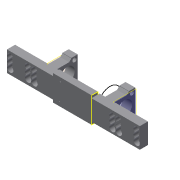
# Autodesk Inventor part: 20_Base_STORMchip_doublesided
Saved by Autodesk Inventor 2019 (Build 230136000, 136)
## iProperties
Created: 2018-09-25
Part Number: 20_Base_STORMchip_doublesided
Material: Generic
Document SubType Name: Modeling
Designer: diederichbenedict
Density: 1 g/cm^3
Appearance: Default
Author: diederichbenedict
Autodesk Inventor part; units mm, degrees
ref_plane "YZ Plane" through (0, 0, 0) normal (1, 0, 0) x (0, 1, 0)
ref_plane "XZ Plane" through (0, 0, 0) normal (0, 1, 0) x (-1, 0, 0)
ref_plane "Work Plane1" through (0, 0, 40) normal (0, 0, 1) x (1, 0, 0)
sketch "Sketch1" plane through (0, 0, 40) normal (0, 0, 1) x (1, 0, 0)
  circle A0 centre (-3.7974, 17.669) radius 1.2295 construction
  line L0 (-20.6474, 15.7142) -> (-23.4129, 15.7142) construction
  arc A1 (-23.4129, 15.7142) -> (-23.682, 15.7142) centre (-23.5474, 13.819) ccw construction
  line L1 (-23.682, 15.7142) -> (-26.0625, 15.7142) construction
  arc A2 (-24.2285, 17.7142) -> (-26.0625, 15.7142) centre (-6.7472, -0.1577) ccw construction
  line L2 (-24.2285, 17.7142) -> (-26.3758, 17.7142) construction
  arc A3 (-26.3758, 17.7142) -> (-24.7023, 19.2398) centre (-27.9474, 21.119) ccw construction
  line L3 (-24.7023, 19.2398) -> (-24.6974, 19.2426) construction
  line L4 (-24.6974, 19.2426) -> (-24.6974, 19.2481) construction
  arc A4 (-24.6974, 19.2481) -> (-24.2285, 20.6377) centre (-27.9474, 21.119) ccw construction
  line L5 (-24.2285, 20.6377) -> (-24.2285, 21.6002) construction
  arc A5 (-24.2285, 21.6002) -> (-24.6974, 22.9898) centre (-27.9474, 21.119) ccw construction
  line L6 (-24.6974, 22.9898) -> (-24.6974, 22.9953) construction
  line L7 (-24.6974, 22.9953) -> (-24.7023, 22.9981) construction
  arc A6 (-24.7023, 22.9981) -> (-24.7753, 23.119) centre (-27.9474, 21.119) ccw construction
  line L8 (-24.2285, 23.119) -> (-24.7753, 23.119) construction
  line L9 (-24.2285, 23.119) -> (-24.2285, 25.119) construction
  line L10 (13.224, 25.119) -> (-24.2285, 25.119) construction
  line L11 (13.224, 15.7142) -> (13.224, 25.119) construction
  line L12 (13.224, 15.7142) -> (24.5758, 15.7142) construction
  line L13 (24.5758, 15.7142) -> (24.5758, 9.2277) construction
  line L14 (24.5758, 9.2277) -> (27.1274, 9.2277) construction
  arc A7 (27.1274, 9.2277) -> (29.8148, 4.5037) centre (29.5758, 7.4941) ccw construction
  line L15 (29.8148, 4.5037) -> (29.8148, 2.9857) construction
  arc A8 (29.8148, 2.9857) -> (29.8148, -2.9952) centre (29.5758, -0.0048) ccw construction
  line L16 (29.8148, -2.9952) -> (29.8148, -5.513) construction
  arc A9 (29.8148, -5.513) -> (27.1391, -10.2535) centre (29.5758, -8.5035) ccw construction
  line L17 (27.1391, -10.2535) -> (24.5758, -10.2535) construction
  line L18 (24.5758, -10.2535) -> (24.5758, -16.281) construction
  line L19 (24.5758, -16.281) -> (13.5758, -16.281) construction
  line L20 (13.5758, -16.281) -> (13.5758, -24.681) construction
  line L21 (-15.9474, -24.681) -> (13.5758, -24.681) construction
  line L22 (-15.9474, -24.681) -> (-15.9474, -23.4032) construction
  arc A10 (-17.9474, -22.5084) -> (-15.9474, -23.4032) centre (-6.7472, -0.1577) ccw construction
  line L23 (-17.9474, -22.5084) -> (-17.9474, -22.681) construction
  line L24 (-24.7753, -22.681) -> (-17.9474, -22.681) construction
  arc A11 (-24.7753, -22.681) -> (-24.7023, -22.5602) centre (-27.9474, -20.681) ccw construction
  line L25 (-24.7023, -22.5602) -> (-24.6974, -22.5574) construction
  line L26 (-24.6974, -22.5574) -> (-24.6974, -22.5519) construction
  arc A12 (-24.6974, -22.5519) -> (-24.6974, -18.8102) centre (-27.9474, -20.681) ccw construction
  line L27 (-24.6974, -18.8102) -> (-24.6974, -18.8047) construction
  line L28 (-24.6974, -18.8047) -> (-24.7023, -18.8019) construction
  arc A13 (-24.7023, -18.8019) -> (-26.3655, -17.281) centre (-27.9474, -20.681) ccw construction
  line L29 (-26.3655, -17.281) -> (-27.3364, -17.281) construction
  line L30 (-27.3364, -17.281) -> (-27.9474, -16.9283) construction
  line L31 (-28.2786, -17.1195) -> (-27.9474, -16.9283) construction
  line L32 (-28.2786, -17.1195) -> (-28.2786, -16.9457) construction
  arc A14 (-28.2786, -16.9457) -> (-29.9474, -17.5089) centre (-27.9474, -20.681) ccw construction
  line L33 (-29.9474, -14.281) -> (-29.9474, -17.5089) construction
  line L34 (-72.9474, -14.281) -> (-29.9474, -14.281) construction
  line L35 (-72.9474, -12.281) -> (-72.9474, -14.281) construction
  arc A15 (-72.9474, -12.281) -> (-66.9474, -4.281) centre (-69.9474, -8.281) ccw construction
  arc A16 (-66.9474, -4.281) -> (-66.9474, 3.719) centre (-69.9474, -0.281) ccw construction
  arc A17 (-66.9474, 3.719) -> (-72.9474, 11.719) centre (-69.9474, 7.719) ccw construction
  line L36 (-72.9474, 13.7142) -> (-72.9474, 11.719) construction
  line L37 (-29.9474, 13.7142) -> (-72.9474, 13.7142) construction
  line L38 (-29.9474, 17.9468) -> (-29.9474, 13.7142) construction
  arc A18 (-29.9474, 17.9468) -> (-28.9474, 17.5047) centre (-27.9474, 21.119) ccw construction
  line L39 (-28.9474, 17.5047) -> (-28.9474, 12.719) construction
  line L40 (-28.9474, 12.719) -> (-28.1759, 12.719) construction
  arc A19 (-26.9474, 14.5715) -> (-28.1759, 12.719) centre (-6.7472, -0.1577) ccw construction
  line L41 (-26.9474, 14.5715) -> (-26.9474, 15.7142) construction
  line L42 (-26.9474, 15.7142) -> (-26.0625, 15.7142) construction
  line L43 (-26.0625, 15.7142) -> (-26.0625, 11.2745) construction
  line L44 (-26.0625, 11.2745) -> (-20.6474, 11.2745) construction
  line L45 (-20.6474, 11.2745) -> (-20.6474, 15.7142) construction
  line L46 (-19.9474, -11.731) -> (-23.1888, -11.731) construction
  arc A20 (-23.1888, -11.731) -> (-25.6444, -11.731) centre (-24.4166, -13.181) ccw construction
  line L47 (-25.6444, -11.731) -> (-27.3166, -11.731) construction
  line L48 (-27.3166, -11.731) -> (-27.3166, -16.481) construction
  line L49 (-27.3166, -16.481) -> (-19.9474, -16.481) construction
  line L50 (-19.9474, -16.481) -> (-19.9474, -11.731) construction
  arc A21 (-24.2786, -17.9803) -> (-22.8499, -19.281) centre (-6.7472, -0.1577) ccw construction
  line L51 (-24.2786, -19.281) -> (-24.2786, -17.9803) construction
  line L52 (-24.2786, -19.281) -> (-22.8499, -19.281) construction
  circle A22 centre (-48.8966, -9.0098) radius 1.45 construction
  circle A23 centre (-62.8966, 8.9902) radius 1.45 construction
  circle A24 centre (-55.8966, -0.0098) radius 1.45 construction
  circle A25 centre (-48.8966, 8.9902) radius 1.45 construction
  circle A26 centre (-62.8966, -9.0098) radius 1.45 construction
  arc A27 (-29.7867, -9.8622) -> (-28.8998, -11.7448) centre (-6.7472, -0.1577) ccw construction
  arc A28 (-29.7867, -9.8622) -> (-31.3026, -4.8512) centre (-31.9474, -7.781) ccw construction
  arc A29 (-31.5545, -3.2552) -> (-31.3026, -4.8512) centre (-6.7472, -0.1577) ccw construction
  arc A30 (-31.5545, -3.2552) -> (-31.5837, 2.6968) centre (-31.9474, -0.281) ccw construction
  arc A31 (-31.1373, 5.3304) -> (-31.5837, 2.6968) centre (-6.7472, -0.1577) ccw construction
  arc A32 (-31.1373, 5.3304) -> (-29.5693, 10.0477) centre (-31.9474, 8.219) ccw construction
  arc A33 (-28.6194, 11.9504) -> (-29.5693, 10.0477) centre (-6.7472, -0.1577) ccw construction
  arc A34 (-28.6194, 11.9504) -> (-36.9474, 8.219) centre (-31.9474, 8.219) ccw construction
  arc A35 (-36.9474, 8.219) -> (-44.5814, 3.969) centre (-41.9474, 8.219) ccw construction
  arc A36 (-44.5814, 3.969) -> (-45.2546, -4.031) centre (-41.9474, -0.281) ccw construction
  arc A37 (-45.2546, -4.031) -> (-36.9474, -7.781) centre (-41.9474, -7.781) ccw construction
  arc A38 (-36.9474, -7.781) -> (-28.8998, -11.7448) centre (-31.9474, -7.781) ccw construction
  line L53 (-19.9474, -11.731) -> (-27.3166, -11.731) construction
  line L54 (-27.3166, -11.731) -> (-27.3166, -16.481) construction
  line L55 (-27.3166, -16.481) -> (-19.9474, -16.481) construction
  line L56 (-19.9474, -16.481) -> (-19.9474, -11.731) construction
  line L57 (-20.6474, 11.2745) -> (-27.3166, 11.2745) construction
  line L58 (-27.3166, 11.2745) -> (-27.3166, 15.7142) construction
  line L59 (-27.3166, 15.7142) -> (-20.6474, 15.7142) construction
  line L60 (-20.6474, 15.7142) -> (-20.6474, 11.2745) construction
  line L61 (-19.9474, -16.481) -> (-27.3166, -16.481)
  line L62 (-27.3166, -16.481) -> (-27.3166, -11.731)
  line L63 (-27.3166, -11.731) -> (-19.9474, -11.731)
  line L64 (-19.9474, -11.731) -> (-19.9474, -16.481)
  line L65 (-20.6474, 11.2745) -> (-27.3166, 11.2745)
  line L66 (-27.3166, 11.2745) -> (-27.3166, 15.7142)
  line L67 (-27.3166, 15.7142) -> (-20.6474, 15.7142)
  line L68 (-20.6474, 15.7142) -> (-20.6474, 11.2745) construction
  circle A39 centre (-24.4166, -13.181) radius 0.6105 projected
  circle A40 centre (-24.4166, -13.181) radius 0.9 projected
  circle A41 centre (-23.5474, 13.819) radius 0.9 projected
  line L69 (-27.3166, -11.731) -> (-21.5681, -11.731)
  line L70 (-21.5681, -11.731) -> (-21.5681, -15.2316)
  line L71 (-21.5681, -15.2316) -> (-27.3166, -15.2316)
  line L72 (-27.3166, -15.2316) -> (-27.3166, -11.731)
  line L73 (-21.5681, 15.7142) -> (-21.5681, 12.3429)
  line L74 (-21.5681, 12.3429) -> (-22.6365, 11.2745)
  point P0 (0, 0)
  dimension "d15" = 135
  constraints: 44 end point, 10 parallel, 6 perpendicular, 5 horizontal, 4 point on line
  measures "d15" angle of L73 L74
extrude "Extrusion1" add sketch "Sketch1" along normal blind 2.0006 contours L62 L63 L70 L71 | L65 L66 L67 L73 L74
sketch "Sketch3" plane through (0, 0, 42.0006) normal (0, 0, 1) x (1, 0, 0)
  line L0 (-26.1307, 11.2745) -> (-26.1307, 15.7142) projected
  line L1 (-26.1307, 15.7142) -> (-19.4616, 15.7142) projected
  line L2 (-19.4616, 15.7142) -> (-19.4616, 11.2745) projected
  line L3 (-19.4616, 11.2745) -> (-26.1307, 11.2745) projected
  line L4 (-18.7616, -11.731) -> (-26.1307, -11.731) projected
  line L5 (-18.7616, -16.481) -> (-18.7616, -11.731) projected
  line L6 (-26.1307, -16.481) -> (-18.7616, -16.481) projected
  line L7 (-26.1307, -11.731) -> (-26.1307, -16.481) projected
  line L8 (-34.5116, -20.2858) -> (-34.5116, 19.7142) projected
  line L9 (25.4884, -20.2858) -> (-34.5116, -20.2858) projected
  line L10 (25.4884, 19.7142) -> (25.4884, -20.2858) projected
  line L11 (-34.5116, 19.7142) -> (25.4884, 19.7142) projected
  circle A0 centre (-24.4166, -13.181) radius 0.9 projected
  circle A1 centre (-23.5474, 13.819) radius 0.9 projected
  point P0 (0, 0)
extrude "Extrusion3" add sketch "Sketch3" along normal blind 10 contours L0 L1 L2 L3 | L5 L6 L7 L4 | L8 L11 L10 L9
sketch "Sketch4" plane through (25.4884, -20.2858, 42.0006) normal (1, 0, 0) x (0, 0, -1)
  line L0 (0, 0) -> (0, 40) projected
  line L1 (0, 40) -> (-10, 40) projected
  line L2 (-10, 0) -> (-10, 40) projected
  line L3 (0, 0) -> (-10, 0) projected
  circle A0 centre (18.7347, 20) radius 17.8578
  point P0 (42.0006, 20.2858)
  constraints: 1 centre point
sketch "Sketch5" plane through (0, 0, 42.0006) normal (0, 0, -1) x (-1, 0, 0)
  circle A0 centre (-22.3026, 2.519) radius 0.6105 projected
  line L0 (-20.5026, 4.519) -> (-24.3026, 4.519) projected
  line L1 (-24.3026, 4.519) -> (-24.3026, -2.881) projected
  line L2 (-24.3026, -2.881) -> (-20.5026, -2.881) projected
  line L3 (-20.5026, -2.881) -> (-20.5026, 4.519) projected
  circle A1 centre (-22.3026, 2.519) radius 0.6105 projected
  line L4 (-20.5026, 5.2475) -> (-24.3026, 5.2475)
  line L5 (-24.3026, 5.2475) -> (-24.3026, 1.4)
  line L6 (-24.3026, 1.4) -> (-20.5026, 1.4)
  line L7 (-20.5026, 1.4) -> (-20.5026, 5.2475)
  point P0 (0, 0)
  constraints: 8 end point, 2 parallel, 1 horizontal, 1 perpendicular, 1 point on line
extrude "Extrusion4" add sketch "Sketch5" along normal blind 3.5 contours L3 L6 L1 L0 | L0 L5 L4 L7
sketch "Sketch7" plane through (0, 0, 52.0006) normal (0, 0, 1) x (1, 0, 0)
  circle A0 centre (68.2852, 7.2142) radius 1 projected
  circle A1 centre (68.2852, -0.2858) radius 1 projected
  circle A2 centre (58.2852, 7.2142) radius 1 projected
  circle A3 centre (96.2852, -8.2858) radius 1 projected
  circle A4 centre (96.2852, -0.2858) radius 1 projected
  circle A5 centre (96.2852, 7.7142) radius 1 projected
  circle A6 centre (58.2852, -0.2858) radius 1 projected
  circle A7 centre (58.2852, -8.7858) radius 1 projected
  circle A8 centre (68.2852, -8.7858) radius 1.0474 projected
  line L0 (101.2852, 15.7142) -> (101.2852, -16.2858) projected
  line L1 (101.2852, 15.7142) -> (53.2852, 15.7142) projected
  line L2 (53.2852, -16.2858) -> (53.2852, 15.7142) projected
  line L3 (101.2852, -16.2858) -> (53.2852, -16.2858) projected
  line L4 (-63.7148, 2.2142) -> (-116.7148, 2.2142)
  circle A9 centre (-73.7148, -7.7858) radius 1 projected
  circle A10 centre (-73.7148, -0.2858) radius 1 projected
  circle A11 centre (-63.7148, -7.7858) radius 1 projected
  circle A12 centre (-101.7148, 7.7142) radius 1 projected
  circle A13 centre (-101.7148, -0.2858) radius 1 projected
  circle A14 centre (-101.7148, -8.2858) radius 1 projected
  circle A15 centre (-63.7148, -0.2858) radius 1 projected
  circle A16 centre (-63.7148, 8.2142) radius 1 projected
  circle A17 centre (-73.7148, 8.2142) radius 1.0474 projected
  line L5 (-106.7148, -16.2858) -> (-106.7148, 15.7142) projected
  line L6 (-106.7148, -16.2858) -> (-58.7148, -16.2858) projected
  line L7 (-58.7148, 15.7142) -> (-58.7148, -16.2858) projected
  line L8 (-106.7148, 15.7142) -> (-58.7148, 15.7142) projected
  line L9 (25.4884, -20.2858) -> (25.4884, 19.7142) projected
  line L10 (101.2852, -16.2858) -> (25.4884, -16.2858)
  line L11 (25.4884, -16.2858) -> (25.4884, 15.7142)
  line L12 (25.4884, 15.7142) -> (101.2852, 15.7142)
  line L13 (101.2852, 15.7142) -> (101.2852, -16.2858)
  line L14 (-34.5116, 19.7142) -> (-34.5116, -20.2858) projected
  line L15 (-106.7148, -16.2858) -> (-34.5116, -16.2858)
  line L16 (-34.5116, -16.2858) -> (-34.5116, 15.7142)
  line L17 (-34.5116, 15.7142) -> (-106.7148, 15.7142)
  line L18 (-106.7148, 15.7142) -> (-106.7148, -16.2858)
  point P0 (0, 0)
  constraints: 18 end point, 4 parallel, 3 horizontal, 3 point on line, 2 perpendicular, 2 other
ref_plane "Work Plane2" through (53.2852, -16.2858, 39.2658) normal (0, 0, 1) x (1, 0, 0)
extrude "Extrusion6" add sketch "Sketch7" against normal up to surface (12.7347 mm away)
ref_plane "Work Plane3" through (49.2852, -0.2858, 23.2658) normal (-1, 0, 0) x (0, 0, 1)
sketch "Sketch8" plane through (49.2852, -0.2858, 23.2658) normal (-1, 0, 0) x (0, 0, 1)
  circle A0 centre (0, 0) radius 6 construction
  line L0 (16, 16) -> (-16, 16) construction
  line L1 (-16, 16) -> (-16, -16) construction
  line L2 (-16, -16) -> (16, -16) construction
  line L3 (16, -16) -> (16, 16) construction
  circle A1 centre (-11.1689, 16.6425) radius 3.2639 construction
  line L4 (-10.0808, -8.1425) -> (-10.0808, 7.3575) projected
  circle A2 centre (-11.1689, -13.3574) radius 3.2639 construction
  circle A3 centre (-11, -15) radius 3.4
  circle A4 centre (-11.1689, 15) radius 3.4
  line L5 (-16, -20) -> (-6.1689, -20)
  line L6 (-6.1689, 20) -> (-16, 20)
  line L7 (-16, 20) -> (-16, -20)
  line L8 (16, -16) -> (-6.1689, -16)
  line L9 (-6.1689, -9.533) -> (-6.1689, 9.533) construction
  line L10 (-6.1689, 16) -> (16, 16)
  line L11 (16, 16) -> (16, -16)
  circle A5 centre (0, 0) radius 11.3549
  line L12 (-6.1689, -20) -> (-6.1689, -16)
  line L13 (-6.1689, 16) -> (-6.1689, 20)
  point P0 (-23.2658, 0.2858)
  dimension "d21" = 6.8
  dimension "d22" = 6.8
  dimension "d23" = 15
  dimension "d24" = 15
  dimension "d25" = 5
  dimension "d26" = 5
  dimension "d27" = 5
  constraints: 18 end point, 5 parallel, 3 centre point, 3 perpendicular, 2 horizontal, 2 point on circle, 2 point on line, 1 coincident
  measures "d21" diameter of A3
  measures "d22" diameter of A4
  measures "d23" vertical distance of A3.centre A0.centre
  measures "d24" vertical distance of A0.centre A4.centre
  measures "d25" distance from line of A3.centre L1
  measures "d26" distance from line of L5 A3.centre
  measures "d27" distance from line of A4.centre L6
extrude "Extrusion7" add sketch "Sketch8" along normal blind 15
ref_plane "Work Plane4" through (-54.7148, -0.2858, 23.2658) normal (1, 0, 0) x (0, 0, 1)
sketch "Sketch9" plane through (-54.7148, -0.2858, 23.2658) normal (1, 0, 0) x (0, 0, 1)
  circle A0 centre (0, 0) radius 11.3549 projected
  circle A1 centre (-11.1689, -15) radius 3.4 projected
  circle A2 centre (-11, 15) radius 3.4 projected
  line L0 (-6.1689, 16) -> (16, 16) projected
  line L1 (16, -16) -> (16, 16) projected
  line L2 (16, -16) -> (-6.1689, -16) projected
  line L3 (-6.1689, -16) -> (-6.1689, -20) projected
  line L4 (-6.1689, -20) -> (-16, -20) projected
  line L5 (-16, -20) -> (-16, 20) projected
  line L6 (-16, 20) -> (-6.1689, 20) projected
  line L7 (-6.1689, 20) -> (-6.1689, 16) projected
  point P0 (-23.2658, -0.2858)
extrude "Extrusion8" add sketch "Sketch9" along normal blind 14
sketch "Sketch10" plane through (0, 0, 52.0006) normal (0, 0, 1) x (1, 0, 0)
  circle A0 centre (-73.7148, -7.7858) radius 1 construction
  circle A1 centre (-73.7148, -0.2858) radius 1 construction
  circle A2 centre (-63.7148, -7.7858) radius 1 construction
  circle A3 centre (-101.7148, 7.7142) radius 1 construction
  circle A4 centre (-101.7148, -0.2858) radius 1 construction
  circle A5 centre (-101.7148, -8.2858) radius 1 construction
  circle A6 centre (-63.7148, -0.2858) radius 1 construction
  circle A7 centre (-63.7148, 8.2142) radius 1 construction
  circle A8 centre (-73.7148, 8.2142) radius 1.0474 construction
  circle A9 centre (68.2852, 7.2142) radius 1 construction
  circle A10 centre (68.2852, -0.2858) radius 1 construction
  circle A11 centre (58.2852, 7.2142) radius 1 construction
  circle A12 centre (96.2852, -8.2858) radius 1 construction
  circle A13 centre (96.2852, -0.2858) radius 1 construction
  circle A14 centre (96.2852, 7.7142) radius 1 construction
  circle A15 centre (58.2852, -0.2858) radius 1 construction
  circle A16 centre (58.2852, -8.7858) radius 1 construction
  circle A17 centre (68.2852, -8.7858) radius 1.0474 construction
  circle A18 centre (-24.4166, -13.181) radius 0.9 construction
  circle A19 centre (-23.5474, 13.819) radius 0.9 construction
  line L0 (-34.5116, 19.7142) -> (-34.5116, 15.7142) construction
  line L1 (-34.5116, 15.7142) -> (-106.7148, 15.7142) construction
  line L2 (-106.7148, 15.7142) -> (-106.7148, -16.2858) construction
  line L3 (-106.7148, -16.2858) -> (-34.5116, -16.2858) construction
  line L4 (-34.5116, -16.2858) -> (-34.5116, -20.2858) construction
  line L5 (-34.5116, -20.2858) -> (25.4884, -20.2858) construction
  line L6 (25.4884, -20.2858) -> (25.4884, -16.2858) construction
  line L7 (25.4884, -16.2858) -> (101.2852, -16.2858) construction
  line L8 (101.2852, -16.2858) -> (101.2852, 15.7142) construction
  line L9 (101.2852, 15.7142) -> (25.4884, 15.7142) construction
  line L10 (25.4884, 15.7142) -> (25.4884, 19.7142) construction
  line L11 (25.4884, 19.7142) -> (-34.5116, 19.7142) construction
  circle A20 centre (68.2852, 7.2142) radius 1 construction
  circle A21 centre (96.2852, -8.2858) radius 1 construction
  point P0 (0, 0)
  point P1 (67.3842, -0.7197)
  constraints: 2 coincident
hole "Hole1" at (58.2852, -8.7858, 52.0006) at (58.2852, -0.2858, 52.0006) at (68.2852, 7.2142, 52.0006) at (67.3842, -0.7197, 52.0006) at (68.2852, -8.7858, 52.0006) at (58.2852, 7.2142, 52.0006) at (96.2852, 7.7142, 52.0006) at (96.2852, -8.2858, 52.0006) at (96.2852, -0.2858, 52.0006) at (-63.7148, -7.7858, 52.0006) at (-73.7148, -7.7858, 52.0006) at (-73.7148, -0.2858, 52.0006) at (-73.7148, 8.2142, 52.0006) at (-63.7148, 8.2142, 52.0006) at (-63.7148, -0.2858, 52.0006) at (-101.7148, -8.2858, 52.0006) at (-101.7148, -0.2858, 52.0006) at (-101.7148, 7.7142, 52.0006) direction (0, 0, -1) diameter 4.5 end through all counterbore diameter 10 counterbore depth 8
chamfer "Chamfer1" distance 3.5 angle 45 4 edges at (41.7852, -16.2858, 17.0969) (-47.7148, -16.2858, 17.0969) (41.7852, 15.7142, 17.0969) (-47.7148, 15.7142, 17.0969)
sketch "Sketch11" plane through (0, 0, 52.0006) normal (0, 0, 1) x (1, 0, 0)
  circle A0 centre (-23.5474, 13.819) radius 0.9 projected
  circle A1 centre (-24.4166, -13.181) radius 0.9 projected
  arc A2 (-60.4076, -4.0358) -> (-61.0809, 3.9642) centre (-63.7148, -0.2858) ccw projected
  arc A3 (-68.7148, -7.7858) -> (-60.4076, -4.0358) centre (-63.7148, -7.7858) ccw projected
  arc A4 (-77.022, -4.0358) -> (-68.7148, -7.7858) centre (-73.7148, -7.7858) ccw projected
  arc A5 (-76.3487, 3.9642) -> (-77.022, -4.0358) centre (-73.7148, -0.2858) ccw projected
  arc A6 (-68.7148, 8.2142) -> (-76.3487, 3.9642) centre (-73.7148, 8.2142) ccw projected
  arc A7 (-61.0809, 3.9642) -> (-68.7148, 8.2142) centre (-63.7148, 8.2142) ccw projected
  arc A8 (63.2852, -8.7858) -> (70.7375, -4.4285) centre (68.2852, -8.7858) ccw projected
  arc A9 (55.6513, -4.5358) -> (63.2852, -8.7858) centre (58.2852, -8.7858) ccw projected
  arc A10 (54.978, 3.4642) -> (55.6513, -4.5358) centre (58.2852, -0.2858) ccw projected
  arc A11 (63.2852, 7.2142) -> (54.978, 3.4642) centre (58.2852, 7.2142) ccw projected
  arc A12 (70.8255, 2.9076) -> (63.2852, 7.2142) centre (68.2852, 7.2142) ccw projected
  arc A13 (70.7375, -4.4285) -> (70.8255, 2.9076) centre (67.3842, -0.7197) ccw projected
  arc A14 (93.2852, -4.2858) -> (101.2852, -8.2858) centre (96.2852, -8.2858) ccw projected
  arc A15 (93.2852, 3.7142) -> (93.2852, -4.2858) centre (96.2852, -0.2858) ccw projected
  arc A16 (101.2852, 7.7142) -> (93.2852, 3.7142) centre (96.2852, 7.7142) ccw projected
  line L0 (101.2852, 7.7142) -> (101.2852, 15.7142) projected
  line L1 (101.2852, 15.7142) -> (25.4884, 15.7142) projected
  line L2 (25.4884, 15.7142) -> (25.4884, 19.7142) projected
  line L3 (25.4884, 19.7142) -> (-34.5116, 19.7142) projected
  line L4 (-34.5116, 19.7142) -> (-34.5116, 15.7142) projected
  line L5 (-34.5116, 15.7142) -> (-106.7148, 15.7142) projected
  line L6 (-106.7148, 15.7142) -> (-106.7148, 7.7142) projected
  arc A17 (-98.7148, 3.7142) -> (-106.7148, 7.7142) centre (-101.7148, 7.7142) ccw projected
  arc A18 (-98.7148, -4.2858) -> (-98.7148, 3.7142) centre (-101.7148, -0.2858) ccw projected
  arc A19 (-106.7148, -8.2858) -> (-98.7148, -4.2858) centre (-101.7148, -8.2858) ccw projected
  line L7 (-106.7148, -8.2858) -> (-106.7148, -16.2858) projected
  line L8 (-106.7148, -16.2858) -> (-34.5116, -16.2858) projected
  line L9 (-34.5116, -16.2858) -> (-34.5116, -20.2858) projected
  line L10 (-34.5116, -20.2858) -> (25.4884, -20.2858) projected
  line L11 (25.4884, -20.2858) -> (25.4884, -16.2858) projected
  line L12 (25.4884, -16.2858) -> (101.2852, -16.2858) projected
  line L13 (101.2852, -16.2858) -> (101.2852, -8.2858) projected
  line L14 (101.2852, 15.7142) -> (101.2852, -16.2858) projected
  line L15 (101.2852, -16.2858) -> (91.2852, -16.2858)
  line L16 (91.2852, -16.2858) -> (91.2852, 15.7142)
  line L17 (91.2852, 15.7142) -> (101.2852, 15.7142)
  line L18 (101.2852, 15.7142) -> (101.2852, -16.2858)
  line L19 (-54.7148, -16.2858) -> (-106.7148, -16.2858) projected
  line L20 (-106.7148, -16.2858) -> (-96.7148, -16.2858)
  line L21 (-96.7148, -16.2858) -> (-96.7148, 15.7142)
  line L22 (-96.7148, 15.7142) -> (-106.7148, 15.7142)
  line L23 (-106.7148, 15.7142) -> (-106.7148, -16.2858)
  point P0 (0, 0)
  constraints: 16 end point, 4 parallel, 2 horizontal, 2 perpendicular, 2 point on line
extrude "Extrusion9" cut sketch "Sketch11" against normal through all contours A15 A16 L14 A14 | A14 L16 A15 | A14 L13 L12 L16 | L16 A16 A15 | L16 L1 L0 A16 | L8 L7 A19 L21 | L21 A17 L6 L5 | A19 L23 A17 A18 | A19 A18 L21 | L21 A18 A17
sketch "Sketch12" plane through (25.4884, -16.2858, 39.2658) normal (0, 0, -1) x (-1, 0, 0)
  line L0 (-8.7968, 32) -> (-8.7968, 0) projected
  line L1 (-8.7968, 0) -> (0, 0) projected
  line L2 (0, 0) -> (0, 32) projected
  line L3 (0, 32) -> (-8.7968, 32) projected
  line L4 (66.2032, 0) -> (66.2032, 32) projected
  line L5 (66.2032, 32) -> (60, 32) projected
  line L6 (60, 32) -> (60, 0) projected
  line L7 (60, 0) -> (66.2032, 0) projected
  line L8 (80.2032, -3.5) -> (66.2032, -3.5) projected
  line L9 (-8.7968, 36.0423) -> (66.2032, 36.0423)
  line L10 (66.2032, 36.0423) -> (66.2032, -3.5)
  line L11 (66.2032, -3.5) -> (-8.7968, -3.5)
  line L12 (-8.7968, -3.5) -> (-8.7968, 36.0423)
  line L13 (66.2032, 36.0423) -> (60, 36.0423)
  line L14 (60, 36.0423) -> (60, -3.5)
  line L15 (60, -3.5) -> (66.2032, -3.5)
  line L16 (66.2032, -3.5) -> (66.2032, 36.0423)
  point P0 (25.4884, 16.2858)
  constraints: 16 end point, 4 parallel, 2 horizontal, 2 perpendicular, 1 point on line
extrude "Extrusion10" cut sketch "Sketch12" against normal up to surface (2.7347 mm away) contours L3 L2 L1 L0 | L5 L4 L7 L6
body "Solid1"
